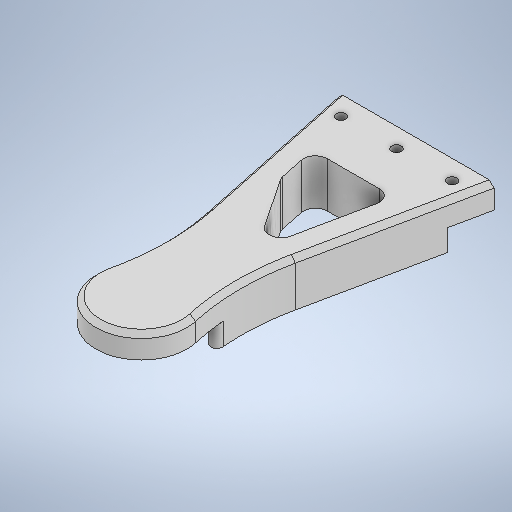
# Autodesk Inventor part: motion_thigh_bot_R
Saved by Autodesk Inventor 2025.2 (Build 292293000, 293)
## iProperties
Created: 2025-04-09
Part Number: motion_thigh_bot_R
Material: Generic
Document SubType Name: Modeling
Designer: Bruno
Density: 1 g/cm^3
Appearance: Default
Mass: 81.6961 g
Surface Area: 177.97 cm^2
Volume: 81.6961 cm^3
Author: Bruno
## iProperties of the stored document motion_thigh_bot_R_3DPrint.ipt
Created: 2025-04-29
Part Number: motion_thigh_bot_R_3DPrint
Material: Generic
Document SubType Name: Modeling
Designer: Bruno
Density: 1 g/cm^3
Appearance: Default
Author: Bruno
Autodesk Inventor part; units mm, degrees
ref_plane "YZ Plane" through (0, 0, 0) normal (1, 0, 0) x (0, 1, 0)
ref_plane "XZ Plane" through (0, 0, 0) normal (0, 1, 0) x (-1, 0, 0)
ref_plane "XY Plane" through (0, 0, 0) normal (0, 0, 1) x (1, 0, 0)
sketch "Sketch1" plane through (0, 0, 0) normal (0, 1, 0) x (-1, 0, 0)
  line L0 (0, 75) -> (0, -75) construction
  arc A0 (18.258988, 69.745538) -> (-18.258988, 69.745538) centre (0, 75) ccw
  line L1 (0, -196.504208) -> (0, 248.158352) construction
  line L2 (-25.341268, -40) -> (25.341268, -40)
  line L3 (25.341268, -40) -> (20, -23.743159)
  line L4 (20, -23.743159) -> (-20, -23.743159)
  line L5 (-20, -23.743159) -> (-25.341268, -40)
  circle A1 centre (12, -31.871075) radius 2
  circle A2 centre (-12, -31.871075) radius 2
  circle A3 centre (0, -31.871075) radius 2
  circle A4 centre (0, -75) radius 23.5
  circle A5 centre (170.873428, 25.827072) radius 158.808057
  circle A6 centre (-170.873428, 25.827072) radius 158.808057
  point P0 (0, 0)
  dimension "d0" = 150
  dimension "d1" = 75
  dimension "d22" = 38
  dimension "d33" = 47
  dimension "d34" = 4
  dimension "d35" = 71.8118
  dimension "d36" = 71.8118
  dimension "d37" = 16.25684
  dimension "d38" = 35
  dimension "d39" = 35
  dimension "d40" = 0
  dimension "d41" = 48.15025
  dimension "d42" = 0
  dimension "d43" = 48.15025
  dimension "d44" = 0
  dimension "d45" = 8.12893
  dimension "d46" = 10.13733
  dimension "d47" = 8.12893
  dimension "d48" = 21.53777
  dimension "d49" = 8.12893
  dimension "d50" = 32.93821
  dimension "d51" = 0
  dimension "d52" = 16.25684
  dimension "d53" = 38.00145
  dimension "d54" = 16.25684
  constraints: 10 end point, 6 centre point, 4 point on circle, 2 coincident, 2 equal radius, 2 tangent, 1 collinear, 1 parallel, 1 point on line, 1 symmetric about line, 1 vertical, 4 other
  measures "d0" distance of L0.start L0.end
  measures "d1" distance of L0.start point (0, 0)
  measures "d22" diameter of A0
  measures "d33" diameter of A4
  measures "d34" diameter of A1
  measures "d35" angle of L2 L3
  measures "d36" angle of L2 L5
  measures "d37" distance between parallel lines of L2 L4
  measures "d38" distance from line of A4.centre L2
  measures "d39" distance from line of A4.centre L5
  measures "d40" distance from line of L2.end L3
  measures "d41" distance from line of L2.end L5
  measures "d42" distance from line of L3.start L2
  measures "d43" distance from line of L2.start L3
  measures "d44" distance from line of L5.end L2
  measures "d45" distance from line of A1.centre L2
  measures "d46" distance from line of A1.centre L3
  measures "d47" distance from line of A3.centre L2
  measures "d48" distance from line of A3.centre L3
  measures "d49" distance from line of A2.centre L2
  measures "d50" distance from line of A2.centre L3
  measures "d51" distance from line of L4.start L3
  measures "d52" distance from line of L3.end L2
  measures "d53" distance from line of L4.end L3
  measures "d54" distance from line of L5.start L2
extrude "Extrusion1" add sketch "Sketch1" along normal blind 10 contours A5 L4 A6 A0 | L3 L2 L5 L4 | A1 | A2
sketch "Sketch4" plane through (0, 10, 0) normal (0, 1, 0) x (1, 0, 0)
  circle A0 centre (3.680608, -72.875) radius 1.5
  circle A1 centre (0, -79.25) radius 1.5
  circle A2 centre (-3.680608, -72.875) radius 1.5
  arc A3 (5.450881, -75.044363) -> (2.76386, -79.69842) centre (10.238345, -80.911111) ccw
  arc A4 (5.450881, -75.044363) -> (2.687021, -70.257217) centre (3.680608, -72.875) ccw
  arc A5 (-2.687021, -70.257217) -> (2.687021, -70.257217) centre (0, -63.177778) ccw
  arc A6 (-2.687021, -70.257217) -> (-5.450881, -75.044363) centre (-3.680608, -72.875) ccw
  arc A7 (-2.76386, -79.69842) -> (-5.450881, -75.044363) centre (-10.238345, -80.911111) ccw
  arc A8 (-2.76386, -79.69842) -> (2.76386, -79.69842) centre (0, -79.25) ccw
  point P0 (0, 0)
extrude "Extrusion4" cut sketch "Sketch4" against normal through all contours A0 | A1 | A2
sketch "Sketch5" plane through (0, 10, 0) normal (0, 1, 0) x (1, 0, 0)
  circle A0 centre (-3.680608, -72.875) radius 1.5
  circle A1 centre (-3.680608, -72.875) radius 2.225
  circle A2 centre (0, -79.25) radius 1.5
  circle A3 centre (0, -79.25) radius 2.225
  circle A4 centre (3.680608, -72.875) radius 1.5
  circle A5 centre (3.680608, -72.875) radius 2.225
  point P0 (0, 0)
  dimension "d69" = 4.45
  dimension "d70" = 4.45
  dimension "d71" = 4.45
  constraints: 3 centre point, 3 coincident
  measures "d69" diameter of A1
  measures "d70" diameter of A3
  measures "d71" diameter of A5
extrude "Extrusion5" cut sketch "Sketch5" against normal blind 6 contours A0 | A1 | A2 | A3 | A4 | A5
sketch "Sketch6" plane through (0, 0, 0) normal (0, -1, 0) x (1, 0, 0)
  circle A0 centre (0, 79.25) radius 1.5
  circle A1 centre (3.680608, 72.875) radius 1.5
  circle A2 centre (-3.680608, 72.875) radius 1.5
  point P0 (0, 0)
extrude "Extrusion6" add sketch "Sketch6" against normal up to surface (4 mm away)
sketch "Sketch7" plane through (0, 0, 0) normal (0, -1, 0) x (1, 0, 0)
  circle A0 centre (23.270461, -31.871075) radius 2
  circle A1 centre (-23.270461, -31.871075) radius 2
  circle A2 centre (0, -31.871075) radius 2
  line L0 (-32.726793, -40) -> (32.726793, -40)
  line L1 (-29.32798, -23.743159) -> (29.32798, -23.743159)
  line L2 (-25.341268, -40) -> (-20, -23.743159)
  line L3 (20, -23.743159) -> (25.341268, -40)
  line L4 (29.32798, -23.743159) -> (32.726793, -40)
  line L5 (-32.726793, -40) -> (-29.32798, -23.743159)
  point P0 (0, 0)
  point P1 (22.130539, -30.227731)
  point P2 (23.327313, -33.870267)
  point P3 (-23.327313, -33.870267)
  point P4 (-22.130539, -30.227731)
extrude "Extrusion7" add sketch "Sketch7" against normal up to surface (10 mm away) contours A0 L3 | A0 L3 L1 L4 L0 | L2 A1 L0 L5 L1 | L2 A1 | A1 L2 picked at (24.149861, -31.36133)
sketch "Sketch8" plane through (0, 10, 0) normal (0, 1, 0) x (1, 0, 0)
  arc A0 (-18.258988, -69.745538) -> (18.258988, -69.745538) centre (0, -75) ccw
  line L0 (0, -75) -> (0, -57.620328) construction
  line L1 (-29.32798, 23.743159) -> (-32.726793, 40)
  line L2 (-29.32798, 23.743159) -> (-18.322098, -28.899016)
  arc A1 (-18.553855, -70.906779) -> (-18.322098, -28.899016) centre (-116.205725, -49.363513) ccw
  arc A2 (-18.258988, -69.745538) -> (18.258988, -69.745538) centre (0, -75) ccw
  circle A3 centre (0, -75) radius 19
  arc A4 (-18.258988, -69.745538) -> (-20, 23.743159) centre (-170.873428, -25.827072) ccw
  line L3 (-20, 23.743159) -> (-29.32798, 23.743159)
  arc A5 (20, 23.743159) -> (18.258988, -69.745538) centre (170.873428, -25.827072) ccw
  line L4 (29.32798, 23.743159) -> (20, 23.743159)
  line L5 (29.32798, 23.743159) -> (18.322098, -28.899016)
  arc A6 (18.322098, -28.899016) -> (18.553855, -70.906779) centre (116.205725, -49.363513) ccw
  point P0 (0, 0)
  point P1 (18.553855, -70.906779)
  point P2 (-18.553855, -70.906779)
  dimension "d80" = 100
  constraints: 6 end point, 4 point on circle, 3 symmetric about line, 2 centre point, 2 tangent, 1 coincident, 1 collinear, 1 vertical, 5 other
  measures "d80" radius of A1
extrude "Extrusion8" add sketch "Sketch8" against normal blind 10 contours A0 A1 L2 L3 A4 | A5 L4 L5 A6 A0
sketch "Sketch11" plane through (0, 0, 0) normal (0, -1, 0) x (1, 0, 0)
  circle A0 centre (23.270461, -31.871075) radius 2
  circle A1 centre (-23.270461, -31.871075) radius 2
  point P0 (0, 0)
extrude "Extrusion11" cut sketch "Sketch11" against normal through all
chamfer "Chamfer1" distance 2 angle 45 5 edges at (-25.5244, 0, -5.5505) (-16.2072, 0, 49.9152) (0, 0, 94) (16.2072, 0, 49.9152) (25.5244, 0, -5.5505)
sketch "Sketch17" plane through (0, 10, 0) normal (0, 1, 0) x (1, 0, 0)
  line L0 (-83.121979, 82.295999) -> (15.75457, -64.379571)
  line L1 (-29.32798, 23.743159) -> (29.32798, 23.743159)
  circle A0 centre (-23.270461, 31.871075) radius 2
  circle A1 centre (23.270461, 31.871075) radius 2
  circle A2 centre (0, 31.871075) radius 2
  arc A3 (-18.553855, -70.906779) -> (18.553855, -70.906779) centre (0, -75) ccw
  arc A4 (18.322098, -28.899016) -> (18.553855, -70.906779) centre (116.205725, -49.363513) ccw
  line L2 (32.726793, 40) -> (18.322098, -28.899016)
  line L3 (-32.726793, 40) -> (32.726793, 40)
  line L4 (-32.726793, 40) -> (-18.322098, -28.899016)
  arc A5 (-18.553855, -70.906779) -> (-18.322098, -28.899016) centre (-116.205725, -49.363513) ccw
  circle A6 centre (-3.680608, -72.875) radius 2.225
  circle A7 centre (0, -79.25) radius 2.225
  circle A8 centre (3.680608, -72.875) radius 2.225
  line L5 (15.75457, -64.379571) -> (17.86641, -67.512319)
  line L6 (-32.726793, 40) -> (-18.322098, -28.899016)
  point P0 (0, 0)
  point P1 (-22.889065, -7.054783)
  constraints: 2 end point, 1 collinear, 1 point on circle
extrude "Extrusion16" add sketch "Sketch17" along normal blind 9 contours L4 L1 L2 A4 L5 L0
sketch "Sketch18" plane through (0, 19, 0) normal (0, 1, 0) x (1, 0, 0)
  circle A0 centre (13.844472, -83.053003) radius 1.5
  circle A1 centre (-8.053003, -88.844472) radius 1.5
  circle A2 centre (8.053003, -61.155528) radius 1.5
  circle A3 centre (-13.844472, -66.946997) radius 1.5
  circle A4 centre (57.038778, -59.914319) radius 1.5
  circle A5 centre (0, -75) radius 12.1825
  line L0 (54.737573, -51.213489) -> (22.535282, -59.730387)
  arc A6 (59.339984, -68.61515) -> (54.737573, -51.213489) centre (57.038778, -59.914319) ccw
  line L1 (27.137693, -77.132048) -> (59.339984, -68.61515)
  arc A7 (27.137693, -77.132048) -> (15.997897, -85.250234) centre (31.995793, -95.500468) ccw
  arc A8 (8.838591, -58.180983) -> (15.997897, -85.250234) centre (0, -75) ccw
  arc A9 (8.838591, -58.180983) -> (22.535282, -59.730387) centre (17.677181, -41.361967) ccw
  arc A10 (18.322098, -28.899016) -> (17.86641, -67.512319) centre (116.205725, -49.363513) ccw
  line L2 (18.322098, -28.899016) -> (29.32798, 23.743159)
  line L3 (29.32798, 23.743159) -> (-29.32798, 23.743159)
  line L4 (-29.32798, 23.743159) -> (-22.889065, -7.054783)
  line L5 (-22.889065, -7.054783) -> (17.86641, -67.512319)
  circle A11 centre (-19.580037, -5.657222) radius 3.525
  circle A12 centre (14.082222, -57.518268) radius 2.448572
  arc A13 (18.322098, -28.899016) -> (17.86641, -67.512319) centre (116.205725, -49.363513) ccw
  point P0 (0, 0)
  point P1 (-22.502925, -7.627592)
  point P2 (-23.030435, -6.378596)
  point P3 (16.523025, -57.323365)
  point P4 (12.051896, -58.886946)
  dimension "d117" = 7.05
  constraints: 5 tangent, 2 centre point
  measures "d117" diameter of A11
extrude "Extrusion17" cut sketch "Sketch18" against normal up to surface (9 mm away) contours A10 L5 A9 | A9 A12 A10 | A9 L5 A12 | L5 L4 A11
sketch "Sketch19" plane through (0, 19, 0) normal (0, 1, 0) x (1, 0, 0)
  arc A0 (-23.030435, -6.378596) -> (-22.502925, -7.627592) centre (-19.580037, -5.657222) ccw
  circle A1 centre (-19.580037, -5.657222) radius 2.225
  circle A2 centre (12.769294, -53.644906) radius 3.525 construction
  line L0 (-22.502925, -7.627592) -> (12.051896, -58.886946)
  arc A3 (18.322098, -28.899016) -> (16.523025, -57.323365) centre (116.205725, -49.363513) ccw
  circle A4 centre (12.769294, -53.644906) radius 2.225
  point P0 (0, 0)
  dimension "d120" = 4.45
  dimension "d121" = 7.05
  dimension "d122" = 4.45
  constraints: 3 centre point, 2 coincident, 2 tangent
  measures "d120" diameter of A1
  measures "d121" diameter of A2
  measures "d122" diameter of A4
extrude "Extrusion18" cut sketch "Sketch19" against normal blind 9.5
sketch "Sketch20" plane through (0, 19, 0) normal (0, 1, 0) x (1, 0, 0)
  circle A0 centre (-19.580037, -5.657222) radius 2.225
  circle A1 centre (12.769294, -53.644906) radius 2.225
  arc A2 (-23.030435, -6.378596) -> (-22.502925, -7.627592) centre (-19.580037, -5.657222) ccw
  line L0 (-22.502925, -7.627592) -> (12.051896, -58.886946)
  arc A3 (12.051896, -58.886946) -> (16.523025, -57.323365) centre (14.082222, -57.518268) ccw
  arc A4 (18.322098, -28.899016) -> (16.523025, -57.323365) centre (116.205725, -49.363513) ccw
  line L1 (18.322098, -28.899016) -> (29.32798, 23.743159)
  line L2 (29.32798, 23.743159) -> (-29.32798, 23.743159)
  line L3 (-29.32798, 23.743159) -> (-23.030435, -6.378596)
  line L4 (-13.501752, -3.090072) -> (7.292792, -33.93714)
  arc A5 (8.533736, -26.852566) -> (7.292792, -33.93714) centre (116.205725, -49.363513) ccw
  line L5 (8.533736, -26.852566) -> (17.02107, 13.743159)
  line L6 (17.02107, 13.743159) -> (-17.02107, 13.743159)
  line L7 (-17.02107, 13.743159) -> (-13.501752, -3.090072)
  point P0 (0, 0)
  dimension "d125" = 10
  constraints: 8 end point, 2 point on circle, 1 centre point, 4 other
  measures "d125" distance between parallel lines of L3 L7
extrude "Extrusion19" cut sketch "Sketch20" against normal through all contours L7 L6 L5 A5 L4
fillet "Fillet2" radius 5 4 edges at (-13.5018, 9.5, 3.0901) (7.2928, 9.5, 33.9371) (-17.0211, 9.5, -13.7432) (17.0211, 9.5, -13.7432)
mirror "Mirror1" about plane through (0, 0, 0) normal (0, 1, 0) remove original yes
sketch "Sketch21" plane through (0, -10, 75) normal (0, -1, 0) x (1, 0, 0)
  line L0 (12.051896, -16.113054) -> (-22.502925, -67.372408)
  arc A0 (16.523025, -17.676635) -> (12.051896, -16.113054) centre (14.082222, -17.481732) ccw
  arc A1 (18.553855, -4.093221) -> (16.523025, -17.676635) centre (116.205725, -25.636487) ccw
  arc A2 (18.553855, -4.093221) -> (-18.553855, -4.093221) centre (0, 0) ccw
  arc A3 (-18.322098, -46.100984) -> (-18.553855, -4.093221) centre (-116.205725, -25.636487) ccw
  line L1 (-23.030435, -68.621404) -> (-18.322098, -46.100984)
  arc A4 (-22.502925, -67.372408) -> (-23.030435, -68.621404) centre (-19.580037, -69.342778) ccw
  circle A5 centre (-3.680608, -2.125) radius 2.225
  circle A6 centre (0, 4.25) radius 2.225
  circle A7 centre (3.680608, -2.125) radius 2.225
  circle A8 centre (0, 0) radius 8.5 construction
  circle A9 centre (0, 0) radius 9.35
  point P0 (0, -75)
  dimension "d129" = 17
  dimension "d130" = 0.85
  constraints: 2 centre point, 2 coincident
  measures "d129" diameter of A8
  measures "d130" radial gap between concentric circles of A9 A8
extrude "Extrusion20" cut sketch "Sketch21" against normal blind 0.2 contours L0 A4 L1 A3 A2 A1 A0
chamfer "Chamfer2" distance 0.2 angle 45 1 edges at (-9.35, -9.8, 75)
equation "\"d1\" = 0.5 * d0"
body "Solid1"
